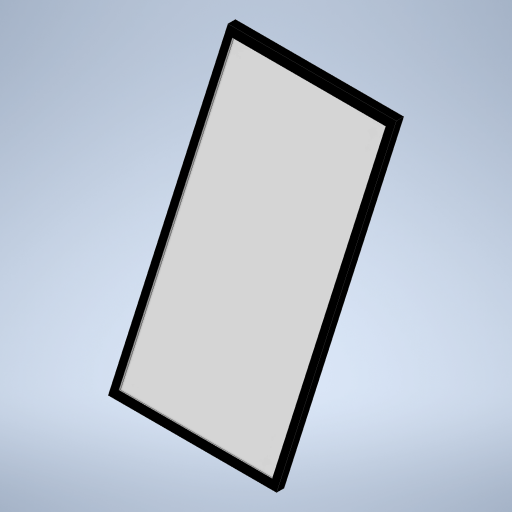
# Autodesk Inventor part: screen
Saved by Autodesk Inventor 2024 (Build 280153000, 153)
## iProperties
Created: 2023-07-16
Part Number: screen
Material: Generic
Document SubType Name: Sheet Metal
Designer: KSABD
Density: 1 g/cm^3
Appearance: Default
Sheet Metal Rule: Default
Author: KSABD
Autodesk Inventor part; units mm, degrees
ref_plane "YZ Plane" through (0, 0, 0) normal (1, 0, 0) x (0, 1, 0)
ref_plane "XZ Plane" through (0, 0, 0) normal (0, 1, 0) x (-1, 0, 0)
ref_plane "XY Plane" through (0, 0, 0) normal (0, 0, 1) x (1, 0, 0)
sketch "Sketch2" plane through (0, 0, 0) normal (1, 0, 0) x (0, 1, 0)
  line L0 (-894.1313, -718.7686) -> (883.8687, -1531.5686)
  line L1 (-894.1313, -667.9686) -> (883.8687, -1480.7686)
  line L2 (-894.1313, -667.9686) -> (883.8687, -667.9686)
  line L3 (-894.1313, -718.7686) -> (-894.1313, -667.9686)
  line L4 (883.8687, -1480.7686) -> (883.8687, -1531.5686)
  point P0 (0, 0)
  dimension "d4" = 1778
  dimension "d5" = 50.8
  dimension "d6" = 50.8
  dimension "d7" = 812.8
  constraints: 10 end point, 2 perpendicular, 1 horizontal
  measures "d4" distance of L1.start L2.end
  measures "d5" distance of L1.start L0.start
  measures "d6" distance of L1.end L0.end
  measures "d7" distance of L2.end L1.end
extrude "Extrusion2" add sketch "Sketch2" along normal blind 1143
sketch "Sketch3" plane through (0, -894.1313, -667.9686) normal (0, 0.4157598, 0.9094745) x (1, 0, 0)
  line L0 (50.8, 1904.1752) -> (1092.2, 1904.1752)
  line L1 (1092.2, 1904.1752) -> (1092.2, 50.8)
  line L2 (1092.2, 50.8) -> (50.8, 50.8)
  line L3 (50.8, 50.8) -> (50.8, 1904.1752)
  line L4 (0, 0) -> (1143, 0) projected
  line L5 (1143, 1954.9752) -> (1143, 0) projected
  line L6 (0, 1954.9752) -> (0, 0) projected
  line L7 (0, 1954.9752) -> (1143, 1954.9752) projected
  point P0 (0, 535.4751)
  dimension "d10" = 50.8
  dimension "d11" = 50.8
  dimension "d12" = 50.8
  dimension "d13" = 50.8
  constraints: 8 end point, 2 parallel, 1 horizontal, 1 perpendicular
  measures "d10" distance between parallel lines of L2 L4
  measures "d11" distance between parallel lines of L5 L1
  measures "d12" distance between parallel lines of L6 L3
  measures "d13" distance between parallel lines of L7 L0
extrude "Extrusion3" cut sketch "Sketch3" against normal blind 12.7 contours L0 L1 L2 L3
equation "\"BendRadius\" = Thickness"
equation "\"BendReliefWidth\" = Thickness"
equation "\"BendReliefDepth\" = 0.5 * Thickness"
equation "\"CornerReliefSize\" = 4 * Thickness"
equation "\"MinimumRemnant\" = 2 * Thickness"
equation "\"TransitionRadius\" = BendRadius"
equation "\"JacobiRadiusSize\" = BendRadius"
equation "\"GapSize\" = Thickness"
equation "\"Thickness\" = 3.048"
body "Solid2"
